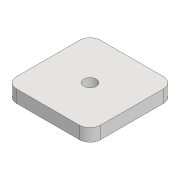
# Autodesk Inventor part: Corpo_2
Saved by Autodesk Inventor 2020 (Build 240168000, 168)
## iProperties
Created: 2022-07-16
Part Number: Corpo_2
Material: Genérico
Document SubType Name: Modeling
Designer: gabri
Density: 1 g/cm^3
Appearance: Padrão
Author: gabri
Autodesk Inventor part; units mm, degrees
ref_plane "YZ Plane" through (0, 0, 0) normal (1, 0, 0) x (0, 1, 0)
ref_plane "XZ Plane" through (0, 0, 0) normal (0, 1, 0) x (-1, 0, 0)
ref_plane "XY Plane" through (0, 0, 0) normal (0, 0, 1) x (1, 0, 0)
sketch "Esboço1" plane through (0, 0, 0) normal (0, 1, 0) x (-1, 0, 0)
  line L0 (0, 0) -> (80, 0)
  line L1 (80, 0) -> (80, -80)
  line L2 (80, -80) -> (0, -80)
  line L3 (0, -80) -> (0, 0)
  circle A0 centre (40, -40) radius 6
  dimension "d0" = 80
  dimension "d1" = 80
  dimension "d2" = 12
  constraints: 8 end point, 2 parallel, 1 centre point, 1 horizontal, 1 perpendicular
  measures "d0" distance of L1.end L2.end
  measures "d1" distance of L0.end L1.end
  measures "d2" diameter of A0
extrude "Extrusão1" add sketch "Esboço1" along normal blind 12
fillet "Arredondamento1" radius 10 4 edges at (-80, 6, 0) (0, 6, 0) (0, 6, -80) (-80, 6, -80)
